Autodesk Inventor part; units mm, degrees
(part 2 of 2)
sketch "FloorSecond_2D" plane through (0, 9, 0) normal (0, 1, 0) x (1, 0, 0)
  line L0 (-96, 71.6) -> (-98, 71.6) projected
  line L1 (-98, 71.6) -> (-98, 4.9) projected
  line L2 (-98, 4.9) -> (-96, 4.9) projected
  line L3 (-96, 4.9) -> (-96, 15) projected
  line L4 (-96, 15) -> (-88, 15) projected
  line L5 (-88, 15) -> (-88, 61.5) projected
  line L6 (-88, 61.5) -> (-96, 61.5) projected
  line L7 (-96, 61.5) -> (-96, 71.6) projected
  line L8 (-95.375, 47.3684) -> (-96.75, 49.75) projected
  line L9 (-96.75, 49.75) -> (-95.375, 52.1316) projected
  line L10 (-95.375, 52.1316) -> (-92.625, 52.1316) projected
  line L11 (-92.625, 52.1316) -> (-91.25, 49.75) projected
  line L12 (-91.25, 49.75) -> (-92.625, 47.3684) projected
  line L13 (-92.625, 47.3684) -> (-95.375, 47.3684) projected
  line L14 (-96.75, 26.75) -> (-95.375, 29.1316) projected
  line L15 (-95.375, 29.1316) -> (-92.625, 29.1316) projected
  line L16 (-92.625, 29.1316) -> (-91.25, 26.75) projected
  line L17 (-91.25, 26.75) -> (-92.625, 24.3684) projected
  line L18 (-92.625, 24.3684) -> (-95.375, 24.3684) projected
  line L19 (-95.375, 24.3684) -> (-96.75, 26.75) projected
  arc A0 (-98, -150) -> (-90, -158) centre (-90, -150) ccw projected
  line L20 (-90, -158) -> (90, -158) projected
  arc A1 (90, -158) -> (98, -150) centre (90, -150) ccw projected
  line L21 (98, -150) -> (98, 150) projected
  arc A2 (98, 150) -> (90, 158) centre (90, 150) ccw projected
  line L22 (90, 158) -> (-90, 158) projected
  arc A3 (-90, 158) -> (-98, 150) centre (-90, 150) ccw projected
  line L23 (-98, 150) -> (-98, 81.4) projected
  line L24 (-98, 81.4) -> (-96, 81.4) projected
  line L25 (-96, 81.4) -> (-96, 91.5) projected
  line L26 (-96, 91.5) -> (-88, 91.5) projected
  line L27 (-88, 91.5) -> (-88, 148) projected
  line L28 (-88, 148) -> (88, 148) projected
  line L29 (88, 148) -> (88, -148) projected
  line L30 (88, -148) -> (-88, -148) projected
  line L31 (-88, -148) -> (-88, -15) projected
  line L32 (-88, -15) -> (-96, -15) projected
  line L33 (-96, -15) -> (-96, -4.9) projected
  line L34 (-96, -4.9) -> (-98, -4.9) projected
  line L35 (-98, -4.9) -> (-98, -150) projected
  line L36 (-1.375, -156.3815) -> (-2.7499, -154) projected
  line L37 (-2.7499, -154) -> (-1.375, -151.6185) projected
  line L38 (-1.375, -151.6185) -> (1.375, -151.6185) projected
  line L39 (1.375, -151.6185) -> (2.7499, -154) projected
  line L40 (2.7499, -154) -> (1.375, -156.3815) projected
  line L41 (1.375, -156.3815) -> (-1.375, -156.3815) projected
  line L42 (91.25, 0) -> (92.625, 2.3816) projected
  line L43 (92.625, 2.3816) -> (95.375, 2.3816) projected
  line L44 (95.375, 2.3816) -> (96.75, 0) projected
  line L45 (96.75, 0) -> (95.375, -2.3816) projected
  line L46 (95.375, -2.3816) -> (92.625, -2.3816) projected
  line L47 (92.625, -2.3816) -> (91.25, 0) projected
  line L48 (-2.7499, 153.5) -> (-1.375, 155.8815) projected
  line L49 (-1.375, 155.8815) -> (1.375, 155.8815) projected
  line L50 (1.375, 155.8815) -> (2.7499, 153.5) projected
  line L51 (2.7499, 153.5) -> (1.375, 151.1185) projected
  line L52 (1.375, 151.1185) -> (-1.375, 151.1185) projected
  line L53 (-1.375, 151.1185) -> (-2.7499, 153.5) projected
  line L54 (-95.375, 100.8684) -> (-96.75, 103.25) projected
  line L55 (-96.75, 103.25) -> (-95.375, 105.6316) projected
  line L56 (-95.375, 105.6316) -> (-92.625, 105.6316) projected
  line L57 (-92.625, 105.6316) -> (-91.25, 103.25) projected
  line L58 (-91.25, 103.25) -> (-92.625, 100.8684) projected
  line L59 (-92.625, 100.8684) -> (-95.375, 100.8684) projected
  line L60 (-96.75, -26.75) -> (-95.375, -24.3684) projected
  line L61 (-95.375, -24.3684) -> (-92.625, -24.3684) projected
  line L62 (-92.625, -24.3684) -> (-91.25, -26.75) projected
  line L63 (-91.25, -26.75) -> (-92.625, -29.1316) projected
  line L64 (-92.625, -29.1316) -> (-95.375, -29.1316) projected
  line L65 (-95.375, -29.1316) -> (-96.75, -26.75) projected
  line L66 (90.6253, -154.3811) -> (89.2505, -152) projected
  line L67 (89.2505, -152) -> (90.6253, -149.6189) projected
  line L68 (90.6253, -149.6189) -> (93.3747, -149.6189) projected
  line L69 (93.3747, -149.6189) -> (94.7495, -152) projected
  line L70 (94.7495, -152) -> (93.3747, -154.3811) projected
  line L71 (93.3747, -154.3811) -> (90.6253, -154.3811) projected
  line L72 (89.2505, 152) -> (90.6253, 154.3811) projected
  line L73 (90.6253, 154.3811) -> (93.3747, 154.3811) projected
  line L74 (93.3747, 154.3811) -> (94.7495, 152) projected
  line L75 (94.7495, 152) -> (93.3747, 149.6189) projected
  line L76 (93.3747, 149.6189) -> (90.6253, 149.6189) projected
  line L77 (90.6253, 149.6189) -> (89.2505, 152) projected
  line L78 (-90.6253, 149.6189) -> (-93.3747, 149.6189) projected
  line L79 (-93.3747, 149.6189) -> (-94.7494, 152) projected
  line L80 (-94.7494, 152) -> (-93.3747, 154.3811) projected
  line L81 (-93.3747, 154.3811) -> (-90.6253, 154.3811) projected
  line L82 (-90.6253, 154.3811) -> (-89.2506, 152) projected
  line L83 (-89.2506, 152) -> (-90.6253, 149.6189) projected
  line L84 (-94.7443, -152) -> (-93.3721, -149.6234) projected
  line L85 (-93.3721, -149.6234) -> (-90.6279, -149.6234) projected
  line L86 (-90.6279, -149.6234) -> (-89.2557, -152) projected
  line L87 (-89.2557, -152) -> (-90.6279, -154.3766) projected
  line L88 (-90.6279, -154.3766) -> (-93.3721, -154.3766) projected
  line L89 (-93.3721, -154.3766) -> (-94.7443, -152) projected
  point P0 (0, 0)
sketch "FloorFirst_2D" plane through (0, 5, 0) normal (0, 1, 0) x (1, 0, 0)
  line L0 (-90, -158) -> (90, -158) projected
  arc A0 (90, -158) -> (98, -150) centre (90, -150) ccw projected
  line L1 (98, -150) -> (98, 150) projected
  arc A1 (98, 150) -> (90, 158) centre (90, 150) ccw projected
  line L2 (90, 158) -> (-90, 158) projected
  arc A2 (-90, 158) -> (-98, 150) centre (-90, 150) ccw projected
  line L3 (-98, 150) -> (-98, -150) projected
  arc A3 (-98, -150) -> (-90, -158) centre (-90, -150) ccw projected
  line L4 (96.75, 0) -> (95.375, -2.3816) projected
  line L5 (95.375, -2.3816) -> (92.625, -2.3816) projected
  line L6 (92.625, -2.3816) -> (91.25, 0) projected
  line L7 (91.25, 0) -> (92.625, 2.3816) projected
  line L8 (92.625, 2.3816) -> (95.375, 2.3816) projected
  line L9 (95.375, 2.3816) -> (96.75, 0) projected
  line L10 (2.7499, 153.5) -> (1.375, 151.1185) projected
  line L11 (1.375, 151.1185) -> (-1.375, 151.1185) projected
  line L12 (-1.375, 151.1185) -> (-2.7499, 153.5) projected
  line L13 (-2.7499, 153.5) -> (-1.375, 155.8815) projected
  line L14 (-1.375, 155.8815) -> (1.375, 155.8815) projected
  line L15 (1.375, 155.8815) -> (2.7499, 153.5) projected
  line L16 (2.7499, -154) -> (1.375, -156.3815) projected
  line L17 (1.375, -156.3815) -> (-1.375, -156.3815) projected
  line L18 (-1.375, -156.3815) -> (-2.7499, -154) projected
  line L19 (-2.7499, -154) -> (-1.375, -151.6185) projected
  line L20 (-1.375, -151.6185) -> (1.375, -151.6185) projected
  line L21 (1.375, -151.6185) -> (2.7499, -154) projected
  line L22 (-91.25, 103.25) -> (-92.625, 100.8684) projected
  line L23 (-92.625, 100.8684) -> (-95.375, 100.8684) projected
  line L24 (-95.375, 100.8684) -> (-96.75, 103.25) projected
  line L25 (-96.75, 103.25) -> (-95.375, 105.6316) projected
  line L26 (-95.375, 105.6316) -> (-92.625, 105.6316) projected
  line L27 (-92.625, 105.6316) -> (-91.25, 103.25) projected
  line L28 (-91.25, 49.75) -> (-92.625, 47.3684) projected
  line L29 (-92.625, 47.3684) -> (-95.375, 47.3684) projected
  line L30 (-95.375, 47.3684) -> (-96.75, 49.75) projected
  line L31 (-96.75, 49.75) -> (-95.375, 52.1316) projected
  line L32 (-95.375, 52.1316) -> (-92.625, 52.1316) projected
  line L33 (-92.625, 52.1316) -> (-91.25, 49.75) projected
  line L34 (-91.25, 26.75) -> (-92.625, 24.3684) projected
  line L35 (-92.625, 24.3684) -> (-95.375, 24.3684) projected
  line L36 (-95.375, 24.3684) -> (-96.75, 26.75) projected
  line L37 (-96.75, 26.75) -> (-95.375, 29.1316) projected
  line L38 (-95.375, 29.1316) -> (-92.625, 29.1316) projected
  line L39 (-92.625, 29.1316) -> (-91.25, 26.75) projected
  line L40 (-91.25, -26.75) -> (-92.625, -29.1316) projected
  line L41 (-92.625, -29.1316) -> (-95.375, -29.1316) projected
  line L42 (-95.375, -29.1316) -> (-96.75, -26.75) projected
  line L43 (-96.75, -26.75) -> (-95.375, -24.3684) projected
  line L44 (-95.375, -24.3684) -> (-92.625, -24.3684) projected
  line L45 (-92.625, -24.3684) -> (-91.25, -26.75) projected
  line L46 (-88, 61.5) -> (-96, 61.5) projected
  line L47 (-96, 61.5) -> (-96, 91.5) projected
  line L48 (-96, 91.5) -> (-88, 91.5) projected
  line L49 (-88, 91.5) -> (-88, 148) projected
  line L50 (-88, 148) -> (88, 148) projected
  line L51 (88, 148) -> (88, -148) projected
  line L52 (88, -148) -> (-88, -148) projected
  line L53 (-88, -148) -> (-88, -15) projected
  line L54 (-88, -15) -> (-96, -15) projected
  line L55 (-96, -15) -> (-96, 15) projected
  line L56 (-96, 15) -> (-88, 15) projected
  line L57 (-88, 15) -> (-88, 61.5) projected
  line L58 (-89.2506, 152) -> (-90.6253, 149.6189) projected
  line L59 (-90.6253, 149.6189) -> (-93.3747, 149.6189) projected
  line L60 (-93.3747, 149.6189) -> (-94.7494, 152) projected
  line L61 (-94.7494, 152) -> (-93.3747, 154.3811) projected
  line L62 (-93.3747, 154.3811) -> (-90.6253, 154.3811) projected
  line L63 (-90.6253, 154.3811) -> (-89.2506, 152) projected
  line L64 (94.7495, 152) -> (93.3747, 149.6189) projected
  line L65 (93.3747, 149.6189) -> (90.6253, 149.6189) projected
  line L66 (90.6253, 149.6189) -> (89.2505, 152) projected
  line L67 (89.2505, 152) -> (90.6253, 154.3811) projected
  line L68 (90.6253, 154.3811) -> (93.3747, 154.3811) projected
  line L69 (93.3747, 154.3811) -> (94.7495, 152) projected
  line L70 (94.7495, -152) -> (93.3747, -154.3811) projected
  line L71 (93.3747, -154.3811) -> (90.6253, -154.3811) projected
  line L72 (90.6253, -154.3811) -> (89.2505, -152) projected
  line L73 (89.2505, -152) -> (90.6253, -149.6189) projected
  line L74 (90.6253, -149.6189) -> (93.3747, -149.6189) projected
  line L75 (93.3747, -149.6189) -> (94.7495, -152) projected
  line L76 (-89.2557, -152) -> (-90.6279, -154.3766) projected
  line L77 (-90.6279, -154.3766) -> (-93.3721, -154.3766) projected
  line L78 (-93.3721, -154.3766) -> (-94.7443, -152) projected
  line L79 (-94.7443, -152) -> (-93.3721, -149.6234) projected
  line L80 (-93.3721, -149.6234) -> (-90.6279, -149.6234) projected
  line L81 (-90.6279, -149.6234) -> (-89.2557, -152) projected
  point P0 (0, 0)
sketch "PCB_2D" plane through (0, 5, 0) normal (0, 1, 0) x (1, 0, 0)
  circle A0 centre (43, -135) radius 1.35 projected
  circle A1 centre (43, 135) radius 1.35 projected
  circle A2 centre (43, -55) radius 1.35 projected
  circle A3 centre (43, 55) radius 1.35 projected
  circle A4 centre (-57.5, -120) radius 1.35 projected
  circle A5 centre (-16, -55) radius 1.35 projected
  circle A6 centre (-16, 55) radius 1.35 projected
  circle A7 centre (-75, -55) radius 1.35 projected
  circle A8 centre (-91.5, 11) radius 1.35 projected
  circle A9 centre (-91.5, 87.5) radius 1.35 projected
  circle A10 centre (-75, 55) radius 1.35 projected
  line L0 (54.9998, -147) -> (54.9998, 147) projected
  line L1 (54.9998, 147) -> (-87, 147) projected
  line L2 (-87, 147) -> (-87, 90.5) projected
  line L3 (-87, 90.5) -> (-96, 90.5) projected
  line L4 (-96, 90.5) -> (-96, 62.5) projected
  line L5 (-96, 62.5) -> (-87, 62.5) projected
  line L6 (-87, 62.5) -> (-87, 14) projected
  line L7 (-87, 14) -> (-96, 14) projected
  line L8 (-96, 14) -> (-96, -14) projected
  line L9 (-96, -14) -> (-87, -14) projected
  line L10 (-87, -14) -> (-87, -147) projected
  line L11 (-87, -147) -> (54.9998, -147) projected
  line L12 (-84.9998, 145.0002) -> (-84.9998, 109.6002) projected
  line L13 (-51.4998, 145.0002) -> (-84.9998, 145.0002) projected
  line L14 (-51.4998, 109.6002) -> (-51.4998, 145.0002) projected
  line L15 (-84.9998, 109.6002) -> (-51.4998, 109.6002) projected
  line L16 (-78.6498, 143.0102) -> (-78.6498, 111.5902) projected
  line L17 (-78.6498, 111.5902) -> (-61.9498, 111.5902) projected
  line L18 (-61.9498, 111.5902) -> (-61.9498, 143.0102) projected
  line L19 (-61.9498, 143.0102) -> (-78.6498, 143.0102) projected
  circle A11 centre (-82.4998, 112.2002) radius 1.5 projected
  circle A12 centre (-82.4998, 142.4002) radius 1.5 projected
  circle A13 centre (-53.9998, 142.4002) radius 1.5 projected
  circle A14 centre (-53.9998, 112.2002) radius 1.5 projected
  line L20 (-84.9998, 127.3002) -> (-82.8998, 127.3002)
  line L21 (-82.8998, 127.3002) -> (-82.8998, 123.4902)
  line L22 (-82.8998, 127.3002) -> (-82.8998, 131.1102)
  circle A15 centre (-82.8998, 123.4902) radius 0.75
  circle A16 centre (-82.8998, 126.0302) radius 0.75
  circle A17 centre (-82.8998, 128.5702) radius 0.75
  circle A18 centre (-82.8998, 131.1102) radius 0.75
  point P0 (0, 0)
  dimension "d370" = 2.1
  dimension "d371" = 3.81
  dimension "d372" = 3.81
  dimension "d373" = 1.5
  dimension "d376" = 2.54
  constraints: 6 end point, 4 centre point, 1 vertical, 6 other
  measures "d370" distance of L20.start L20.end
  measures "d371" distance of L21.start L21.end
  measures "d372" distance of L22.start L22.end
  measures "d373" diameter of A15
  measures "d376" distance of A15.centre A16.centre
